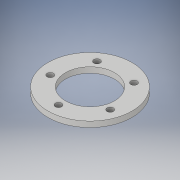
# Autodesk Inventor part: wheel-drill-template
Saved by Autodesk Inventor 2018 (Build 220112000, 112)
## iProperties
Created: 2017-10-19
Part Number: wheel-drill-template
Material: Generic
Document SubType Name: Modeling
Designer: leo2a
Density: 1 g/cm^3
Appearance: Default
Author: leo2a
Autodesk Inventor part; units mm, degrees
ref_plane "YZ Plane" through (0, 0, 0) normal (1, 0, 0) x (0, 1, 0)
ref_plane "XZ Plane" through (0, 0, 0) normal (0, 1, 0) x (-1, 0, 0)
ref_plane "XY Plane" through (0, 0, 0) normal (0, 0, 1) x (1, 0, 0)
sketch "Sketch1" plane through (0, 0, 0) normal (0, 1, 0) x (-1, 0, 0)
  circle A0 centre (0, 0) radius 19.05
  circle A1 centre (0, 0) radius 11.1125
  dimension "d0" = 38.1
  dimension "d1" = 22.225
  constraints: 2 centre point, 2 coincident
  measures "d0" diameter of A0
  measures "d1" diameter of A1
extrude "Extrusion1" add sketch "Sketch1" along normal blind 2.54
sketch "Sketch2" plane through (0, 2.54, 0) normal (0, 1, 0) x (1, 0, 0)
  line L0 (0, 0) -> (0, -14.2875)
  line L1 (0, -14.2875) -> (-13.5882, -4.4151)
  line L2 (-13.5882, -4.4151) -> (-8.398, 11.5588)
  line L3 (-8.398, 11.5588) -> (8.398, 11.5588)
  line L4 (8.398, 11.5588) -> (13.5882, -4.4151)
  line L5 (13.5882, -4.4151) -> (0, -14.2875)
  dimension "d4" = 14.2875
  constraints: 12 end point, 6 coincident, 1 vertical, 11 other
  measures "d4" distance of L0.start L0.end
hole "Hole1" at (0, 2.54, 14.2875) at (-13.5882, 2.54, 4.4151) at (-8.398, 2.54, -11.5588) at (8.398, 2.54, -11.5588) at (13.5882, 2.54, 4.4151) direction (0, -1, 0) diameter 2.8956 end through all clearance for "Socket Head Cap Screw ISO 4762" size "M2.5" standard "ISO"
body "Solid1"
